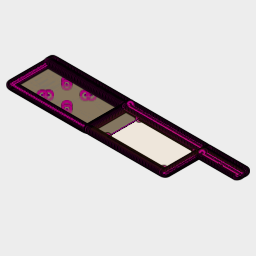
Case v2 (Autodesk Fusion 360 design; units mm, degrees)
Autodesk Fusion 360 part; units mm, degrees
(part 1 of 8)
sketch "Sketch4" plane through (0, 0, 0) normal (0, 1, 0) x (1, 0, 0)
  line L0 (6.35, -6.35) -> (11.1, -6.35)
  line L1 (11.1, -6.35) -> (11.1, -9.35)
  line L2 (11.1, -9.35) -> (15.85, -9.35)
  line L3 (15.85, -9.35) -> (15.85, -6.35)
  line L4 (15.85, -6.35) -> (18.85, -6.35)
  line L5 (18.85, -6.35) -> (18.85, -9.35)
  line L6 (18.85, -9.35) -> (21.85, -9.35)
  line L7 (21.85, -9.35) -> (21.85, -6.35)
  line L8 (21.85, -6.35) -> (24.85, -6.35)
  line L9 (24.85, -6.35) -> (24.85, -9.35)
  line L10 (24.85, -9.35) -> (27.85, -9.35)
  line L11 (27.85, -9.35) -> (27.85, -6.35)
  line L12 (27.85, -6.35) -> (30.85, -6.35)
  line L13 (30.85, -6.35) -> (30.85, -9.35)
  line L14 (30.85, -9.35) -> (33.85, -9.35)
  line L15 (33.85, -9.35) -> (33.85, -6.35)
  line L16 (33.85, -6.35) -> (36.85, -6.35)
  line L17 (36.85, -6.35) -> (36.85, -9.35)
  line L18 (36.85, -9.35) -> (39.85, -9.35)
  line L19 (39.85, -9.35) -> (39.85, -6.35)
  line L20 (39.85, -6.35) -> (42.85, -6.35)
  line L21 (42.85, -6.35) -> (42.85, -9.35)
  line L22 (42.85, -9.35) -> (45.85, -9.35)
  line L23 (45.85, -9.35) -> (45.85, -6.35)
  line L24 (45.85, -6.35) -> (48.85, -6.35)
  line L25 (48.85, -6.35) -> (48.85, -9.35)
  line L26 (48.85, -9.35) -> (51.85, -9.35)
  line L27 (51.85, -9.35) -> (51.85, -6.35)
  line L28 (51.85, -6.35) -> (54.85, -6.35)
  line L29 (54.85, -6.35) -> (54.85, -9.35)
  line L30 (54.85, -9.35) -> (57.85, -9.35)
  line L31 (57.85, -9.35) -> (57.85, -6.35)
  line L32 (57.85, -6.35) -> (60.8501, -6.35)
  line L33 (60.8501, -6.35) -> (60.8501, -9.35)
  line L34 (60.8501, -9.35) -> (63.8501, -9.35)
  line L35 (63.8501, -9.35) -> (63.8501, -6.35)
  line L36 (63.8501, -6.35) -> (66.8501, -6.35)
  line L37 (66.8501, -6.35) -> (66.8501, -9.35)
  line L38 (66.8501, -9.35) -> (69.8501, -9.35)
  line L39 (69.8501, -9.35) -> (69.8501, -6.35)
  line L40 (69.8501, -6.35) -> (72.8501, -6.35)
  line L41 (72.8501, -6.35) -> (72.8501, -9.35)
  line L42 (72.8501, -9.35) -> (75.8501, -9.35)
  line L43 (75.8501, -9.35) -> (75.8501, -6.35)
  line L44 (75.8501, -6.35) -> (78.8501, -6.35)
  line L45 (78.8501, -6.35) -> (78.8501, -9.35)
  line L46 (78.8501, -9.35) -> (81.8501, -9.35)
  line L47 (81.8501, -9.35) -> (81.8501, -6.35)
  line L48 (81.8501, -6.35) -> (84.8501, -6.35)
  line L49 (84.8501, -6.35) -> (84.8501, -9.35)
  line L50 (84.8501, -9.35) -> (87.8501, -9.35)
  line L51 (87.8501, -9.35) -> (87.8501, -6.35)
  line L52 (87.8501, -6.35) -> (90.8501, -6.35)
  line L53 (90.8501, -6.35) -> (90.8501, -9.35)
  line L54 (90.8501, -9.35) -> (93.8501, -9.35)
  line L55 (93.8501, -9.35) -> (93.8501, -6.35)
  line L56 (93.8501, -6.35) -> (96.8501, -6.35)
  line L57 (96.8501, -6.35) -> (96.8501, -9.35)
  line L58 (96.8501, -9.35) -> (99.8501, -9.35)
  line L59 (99.8501, -9.35) -> (99.8501, -6.35)
  line L60 (99.8501, -6.35) -> (102.8501, -6.35)
  line L61 (102.8501, -6.35) -> (102.8501, -9.35)
  line L62 (102.8501, -9.35) -> (105.8501, -9.35)
  line L63 (105.8501, -9.35) -> (105.8501, -6.35)
  line L64 (105.8501, -6.35) -> (108.8501, -6.35)
  line L65 (108.8501, -6.35) -> (108.8501, -9.35)
  line L66 (108.8501, -9.35) -> (111.8501, -9.35)
  line L67 (111.8501, -9.35) -> (111.8501, -6.35)
  line L68 (111.8501, -6.35) -> (114.8501, -6.35)
  line L69 (114.8501, -6.35) -> (114.8501, -9.35)
  line L70 (114.8501, -9.35) -> (117.8501, -9.35)
  line L71 (117.8501, -9.35) -> (117.8501, -6.35)
  line L72 (117.8501, -6.35) -> (120.8501, -6.35)
  line L73 (120.8501, -6.35) -> (120.8501, -9.35)
  line L74 (120.8501, -9.35) -> (123.8501, -9.35)
  line L75 (123.8501, -9.35) -> (123.8501, -6.35)
  line L76 (123.8501, -6.35) -> (126.8501, -6.35)
  line L77 (126.8501, -6.35) -> (126.8501, -9.35)
  line L78 (126.8501, -9.35) -> (129.8501, -9.35)
  line L79 (129.8501, -9.35) -> (129.8501, -6.35)
  line L80 (129.8501, -6.35) -> (132.8501, -6.35)
  line L81 (132.8501, -6.35) -> (132.8501, -9.35)
  line L82 (132.8501, -9.35) -> (135.8501, -9.35)
  line L83 (135.8501, -9.35) -> (135.8501, -6.35)
  line L84 (135.8501, -6.35) -> (138.8501, -6.35)
  line L85 (138.8501, -6.35) -> (138.8501, -9.35)
  line L86 (138.8501, -9.35) -> (141.8501, -9.35)
  line L87 (141.8501, -9.35) -> (141.8501, -6.35)
  line L88 (141.8501, -6.35) -> (144.8501, -6.35)
  line L89 (144.8501, -6.35) -> (144.8501, -9.35)
  line L90 (144.8501, -9.35) -> (147.8501, -9.35)
  line L91 (147.8501, -9.35) -> (147.8501, -6.35)
  line L92 (147.8501, -6.35) -> (150.8501, -6.35)
  line L93 (150.8501, -6.35) -> (150.8501, -9.35)
  line L94 (150.8501, -9.35) -> (153.8501, -9.35)
  line L95 (153.8501, -9.35) -> (153.8501, -6.35)
  line L96 (153.8501, -6.35) -> (156.8501, -6.35)
  line L97 (156.8501, -6.35) -> (156.8501, -9.35)
  line L98 (156.8501, -9.35) -> (159.8501, -9.35)
  line L99 (159.8501, -9.35) -> (159.8501, -6.35)
  line L100 (159.8501, -6.35) -> (162.8501, -6.35)
  line L101 (162.8501, -6.35) -> (162.8501, -9.35)
  line L102 (162.8501, -9.35) -> (165.8501, -9.35)
  line L103 (165.8501, -9.35) -> (165.8501, -6.35)
  line L104 (165.8501, -6.35) -> (168.8501, -6.35)
  line L105 (168.8501, -6.35) -> (168.8501, -9.35)
  line L106 (168.8501, -9.35) -> (171.8501, -9.35)
  line L107 (171.8501, -9.35) -> (171.8501, -6.35)
  line L108 (171.8501, -6.35) -> (174.8501, -6.35)
  line L109 (174.8501, -6.35) -> (174.8501, -9.35)
  line L110 (174.8501, -9.35) -> (177.8501, -9.35)
  line L111 (177.8501, -9.35) -> (177.8501, -6.35)
  line L112 (177.8501, -6.35) -> (180.8501, -6.35)
  line L113 (180.8501, -6.35) -> (180.8501, -9.35)
  line L114 (180.8501, -9.35) -> (183.8502, -9.35)
  line L115 (183.8502, -9.35) -> (183.8502, -6.35)
  line L116 (183.8502, -6.35) -> (186.8502, -6.35)
  line L117 (186.8502, -6.35) -> (186.8502, -9.35)
  line L118 (186.8502, -9.35) -> (189.8502, -9.35)
  line L119 (189.8502, -9.35) -> (189.8502, -6.35)
  line L120 (189.8502, -6.35) -> (192.8502, -6.35)
  line L121 (192.8502, -6.35) -> (192.8502, -9.35)
  line L122 (192.8502, -9.35) -> (195.8502, -9.35)
  line L123 (195.8502, -9.35) -> (195.8502, -6.35)
  line L124 (195.8502, -6.35) -> (198.8502, -6.35)
  line L125 (198.8502, -6.35) -> (198.8502, -9.35)
  line L126 (198.8502, -9.35) -> (201.8502, -9.35)
  line L127 (201.8502, -9.35) -> (201.8502, -6.35)
  line L128 (201.8502, -6.35) -> (204.8502, -6.35)
  line L129 (204.8502, -6.35) -> (204.8502, -9.35)
  line L130 (204.8502, -9.35) -> (207.8502, -9.35)
  line L131 (207.8502, -9.35) -> (207.8502, -6.35)
  line L132 (207.8502, -6.35) -> (210.8502, -6.35)
  line L133 (210.8502, -6.35) -> (210.8502, -9.35)
  line L134 (210.8502, -9.35) -> (213.8502, -9.35)
  line L135 (213.8502, -9.35) -> (213.8502, -6.35)
  line L136 (213.8502, -6.35) -> (216.8502, -6.35)
  line L137 (216.8502, -6.35) -> (216.8502, -9.35)
  line L138 (216.8502, -9.35) -> (219.8502, -9.35)
  line L139 (219.8502, -9.35) -> (219.8502, -6.35)
  line L140 (219.8502, -6.35) -> (222.8502, -6.35)
  line L141 (222.8502, -6.35) -> (222.8502, -9.35)
  line L142 (222.8502, -9.35) -> (225.8502, -9.35)
  line L143 (225.8502, -9.35) -> (225.8502, -6.35)
  line L144 (225.8502, -6.35) -> (228.8502, -6.35)
  line L145 (228.8502, -6.35) -> (228.8502, -9.35)
  line L146 (228.8502, -9.35) -> (231.8502, -9.35)
  line L147 (231.8502, -9.35) -> (231.8502, -6.35)
  line L148 (231.8502, -6.35) -> (234.8502, -6.35)
  line L149 (234.8502, -6.35) -> (234.8502, -9.35)
  line L150 (234.8502, -9.35) -> (237.8502, -9.35)
  line L151 (237.8502, -9.35) -> (237.8502, -6.35)
  line L152 (237.8502, -6.35) -> (240.8502, -6.35)
  line L153 (240.8502, -6.35) -> (240.8502, -9.35)
  line L154 (240.8502, -9.35) -> (243.8502, -9.35)
  line L155 (243.8502, -9.35) -> (243.8502, -6.35)
  line L156 (243.8502, -6.35) -> (246.8502, -6.35)
  line L157 (246.8502, -6.35) -> (246.8502, -9.35)
  line L158 (246.8502, -9.35) -> (249.8502, -9.35)
  line L159 (249.8502, -9.35) -> (249.8502, -6.35)
  line L160 (249.8502, -6.35) -> (252.8502, -6.35)
  line L161 (252.8502, -6.35) -> (252.8502, -9.35)
  line L162 (252.8502, -9.35) -> (255.8502, -9.35)
  line L163 (255.8502, -9.35) -> (255.8502, -6.35)
  line L164 (255.8502, -6.35) -> (258.8502, -6.35)
  line L165 (258.8502, -6.35) -> (258.8502, -9.35)
  line L166 (258.8502, -9.35) -> (261.8502, -9.35)
  line L167 (261.8502, -9.35) -> (261.8502, -6.35)
  line L168 (261.8502, -6.35) -> (264.8502, -6.35)
  line L169 (264.8502, -6.35) -> (264.8502, -9.35)
  line L170 (264.8502, -9.35) -> (267.8502, -9.35)
  line L171 (267.8502, -9.35) -> (267.8502, -6.35)
  line L172 (267.8502, -6.35) -> (270.8502, -6.35)
  line L173 (270.8502, -6.35) -> (270.8502, -9.35)
  line L174 (270.8502, -9.35) -> (273.8502, -9.35)
  line L175 (273.8502, -9.35) -> (273.8502, -6.35)
  line L176 (273.8502, -6.35) -> (276.8502, -6.35)
  line L177 (276.8502, -6.35) -> (276.8502, -9.35)
  line L178 (276.8502, -9.35) -> (279.8502, -9.35)
  line L179 (279.8502, -9.35) -> (279.8502, -6.35)
  line L180 (279.8502, -6.35) -> (282.8502, -6.35)
  line L181 (282.8502, -6.35) -> (282.8502, -9.35)
  line L182 (282.8502, -9.35) -> (285.8502, -9.35)
  line L183 (285.8502, -9.35) -> (285.8502, -6.35)
  line L184 (285.8502, -6.35) -> (288.8502, -6.35)
  line L185 (288.8502, -6.35) -> (288.8502, -9.35)
  line L186 (288.8502, -9.35) -> (291.8502, -9.35)
  line L187 (291.8502, -9.35) -> (291.8502, -6.35)
  line L188 (291.8502, -6.35) -> (294.8502, -6.35)
  line L189 (294.8502, -6.35) -> (294.8502, -9.35)
  line L190 (294.8502, -9.35) -> (297.8502, -9.35)
  line L191 (297.8502, -9.35) -> (297.8502, -6.35)
  line L192 (297.8502, -6.35) -> (300.8502, -6.35)
  line L193 (300.8502, -6.35) -> (300.8502, -9.35)
  line L194 (300.8502, -9.35) -> (303.8502, -9.35)
  line L195 (303.8502, -9.35) -> (303.8502, -6.35)
  line L196 (303.8502, -6.35) -> (306.8503, -6.35)
  line L197 (306.8503, -6.35) -> (306.8503, -9.35)
  line L198 (306.8503, -9.35) -> (309.8503, -9.35)
  line L199 (309.8503, -9.35) -> (309.8503, -6.35)
  line L200 (309.8503, -6.35) -> (312.8503, -6.35)
  line L201 (312.8503, -6.35) -> (312.8503, -9.35)
  line L202 (312.8503, -9.35) -> (317.6003, -9.35)
  line L203 (317.6003, -9.35) -> (317.6003, -6.35)
  line L204 (317.6003, -6.35) -> (322.3503, -6.35)
  line L205 (322.3503, -6.35) -> (322.3503, -10.1)
  line L206 (322.3503, -10.1) -> (319.3503, -10.1)
  line L207 (319.3503, -10.1) -> (319.3503, -13.85)
  line L208 (319.3503, -13.85) -> (322.3503, -13.85)
  line L209 (322.3503, -13.85) -> (322.3503, -16.85)
  line L210 (322.3503, -16.85) -> (319.3503, -16.85)
  line L211 (319.3503, -16.85) -> (319.3503, -20.6)
  line L212 (319.3503, -20.6) -> (322.3503, -20.6)
  line L213 (322.3503, -20.6) -> (322.3503, -24.35)
  line L214 (322.3503, -24.35) -> (317.6003, -24.35)
  line L215 (317.6003, -24.35) -> (317.6003, -21.35)
  line L216 (317.6003, -21.35) -> (312.8503, -21.35)
  line L217 (312.8503, -21.35) -> (312.8503, -24.35)
  line L218 (312.8503, -24.35) -> (309.8503, -24.35)
  line L219 (309.8503, -24.35) -> (309.8503, -21.35)
  line L220 (309.8503, -21.35) -> (306.8503, -21.35)
  line L221 (306.8503, -21.35) -> (306.8503, -24.35)
  line L222 (306.8503, -24.35) -> (303.8502, -24.35)
  line L223 (303.8502, -24.35) -> (303.8502, -21.35)
  line L224 (303.8502, -21.35) -> (300.8502, -21.35)
  line L225 (300.8502, -21.35) -> (300.8502, -24.35)
  line L226 (300.8502, -24.35) -> (297.8502, -24.35)
  line L227 (297.8502, -24.35) -> (297.8502, -21.35)
  line L228 (297.8502, -21.35) -> (294.8502, -21.35)
  line L229 (294.8502, -21.35) -> (294.8502, -24.35)
  line L230 (294.8502, -24.35) -> (291.8502, -24.35)
  line L231 (291.8502, -24.35) -> (291.8502, -21.35)
  line L232 (291.8502, -21.35) -> (288.8502, -21.35)
  line L233 (288.8502, -21.35) -> (288.8502, -24.35)
  line L234 (288.8502, -24.35) -> (285.8502, -24.35)
  line L235 (285.8502, -24.35) -> (285.8502, -21.35)
  line L236 (285.8502, -21.35) -> (282.8502, -21.35)
  line L237 (282.8502, -21.35) -> (282.8502, -24.35)
  line L238 (282.8502, -24.35) -> (279.8502, -24.35)
  line L239 (279.8502, -24.35) -> (279.8502, -21.35)
  line L240 (279.8502, -21.35) -> (276.8502, -21.35)
  line L241 (276.8502, -21.35) -> (276.8502, -24.35)
  line L242 (276.8502, -24.35) -> (273.8502, -24.35)
  line L243 (273.8502, -24.35) -> (273.8502, -21.35)
  line L244 (273.8502, -21.35) -> (270.8502, -21.35)
  line L245 (270.8502, -21.35) -> (270.8502, -24.35)
  line L246 (270.8502, -24.35) -> (267.8502, -24.35)
  line L247 (267.8502, -24.35) -> (267.8502, -21.35)
  line L248 (267.8502, -21.35) -> (264.8502, -21.35)
  line L249 (264.8502, -21.35) -> (264.8502, -24.35)
  line L250 (264.8502, -24.35) -> (261.8502, -24.35)
  line L251 (261.8502, -24.35) -> (261.8502, -21.35)
  line L252 (261.8502, -21.35) -> (258.8502, -21.35)
  line L253 (258.8502, -21.35) -> (258.8502, -24.35)
  line L254 (258.8502, -24.35) -> (255.8502, -24.35)
  line L255 (255.8502, -24.35) -> (255.8502, -21.35)
  line L256 (255.8502, -21.35) -> (252.8502, -21.35)
  line L257 (252.8502, -21.35) -> (252.8502, -24.35)
  line L258 (252.8502, -24.35) -> (249.8502, -24.35)
  line L259 (249.8502, -24.35) -> (249.8502, -21.35)
  line L260 (249.8502, -21.35) -> (246.8502, -21.35)
  line L261 (246.8502, -21.35) -> (246.8502, -24.35)
  line L262 (246.8502, -24.35) -> (243.8502, -24.35)
  line L263 (243.8502, -24.35) -> (243.8502, -21.35)
  line L264 (243.8502, -21.35) -> (240.8502, -21.35)
  line L265 (240.8502, -21.35) -> (240.8502, -24.35)
  line L266 (240.8502, -24.35) -> (237.8502, -24.35)
  line L267 (237.8502, -24.35) -> (237.8502, -21.35)
  line L268 (237.8502, -21.35) -> (234.8502, -21.35)
  line L269 (234.8502, -21.35) -> (234.8502, -24.35)
  line L270 (234.8502, -24.35) -> (231.8502, -24.35)
  line L271 (231.8502, -24.35) -> (231.8502, -21.35)
  line L272 (231.8502, -21.35) -> (228.8502, -21.35)
  line L273 (228.8502, -21.35) -> (228.8502, -24.35)
  line L274 (228.8502, -24.35) -> (225.8502, -24.35)
  line L275 (225.8502, -24.35) -> (225.8502, -21.35)
  line L276 (225.8502, -21.35) -> (222.8502, -21.35)
  line L277 (222.8502, -21.35) -> (222.8502, -24.35)
  line L278 (222.8502, -24.35) -> (219.8502, -24.35)
  line L279 (219.8502, -24.35) -> (219.8502, -21.35)
  line L280 (219.8502, -21.35) -> (216.8502, -21.35)
  line L281 (216.8502, -21.35) -> (216.8502, -24.35)
  line L282 (216.8502, -24.35) -> (213.8502, -24.35)
  line L283 (213.8502, -24.35) -> (213.8502, -21.35)
  line L284 (213.8502, -21.35) -> (210.8502, -21.35)
  line L285 (210.8502, -21.35) -> (210.8502, -24.35)
  line L286 (210.8502, -24.35) -> (207.8502, -24.35)
  line L287 (207.8502, -24.35) -> (207.8502, -21.35)
  line L288 (207.8502, -21.35) -> (204.8502, -21.35)
  line L289 (204.8502, -21.35) -> (204.8502, -24.35)
  line L290 (204.8502, -24.35) -> (201.8502, -24.35)
  line L291 (201.8502, -24.35) -> (201.8502, -21.35)
  line L292 (201.8502, -21.35) -> (198.8502, -21.35)
  line L293 (198.8502, -21.35) -> (198.8502, -24.35)
  line L294 (198.8502, -24.35) -> (195.8502, -24.35)
  line L295 (195.8502, -24.35) -> (195.8502, -21.35)
  line L296 (195.8502, -21.35) -> (192.8502, -21.35)
  line L297 (192.8502, -21.35) -> (192.8502, -24.35)
  line L298 (192.8502, -24.35) -> (189.8502, -24.35)
  line L299 (189.8502, -24.35) -> (189.8502, -21.35)
  line L300 (189.8502, -21.35) -> (186.8502, -21.35)
  line L301 (186.8502, -21.35) -> (186.8502, -24.35)
  line L302 (186.8502, -24.35) -> (183.8502, -24.35)
  line L303 (183.8502, -24.35) -> (183.8502, -21.35)
  line L304 (183.8502, -21.35) -> (180.8501, -21.35)
  line L305 (180.8501, -21.35) -> (180.8501, -24.35)
  line L306 (180.8501, -24.35) -> (177.8501, -24.35)
  line L307 (177.8501, -24.35) -> (177.8501, -21.35)
  line L308 (177.8501, -21.35) -> (174.8501, -21.35)
  line L309 (174.8501, -21.35) -> (174.8501, -24.35)
  line L310 (174.8501, -24.35) -> (171.8501, -24.35)
  line L311 (171.8501, -24.35) -> (171.8501, -21.35)
  line L312 (171.8501, -21.35) -> (168.8501, -21.35)
  line L313 (168.8501, -21.35) -> (168.8501, -24.35)
  line L314 (168.8501, -24.35) -> (165.8501, -24.35)
  line L315 (165.8501, -24.35) -> (165.8501, -21.35)
  line L316 (165.8501, -21.35) -> (162.8501, -21.35)
  line L317 (162.8501, -21.35) -> (162.8501, -24.35)
  line L318 (162.8501, -24.35) -> (159.8501, -24.35)
  line L319 (159.8501, -24.35) -> (159.8501, -21.35)
  line L320 (159.8501, -21.35) -> (156.8501, -21.35)
  line L321 (156.8501, -21.35) -> (156.8501, -24.35)
  line L322 (156.8501, -24.35) -> (153.8501, -24.35)
  line L323 (153.8501, -24.35) -> (153.8501, -21.35)
  line L324 (153.8501, -21.35) -> (150.8501, -21.35)
  line L325 (150.8501, -21.35) -> (150.8501, -24.35)
  line L326 (150.8501, -24.35) -> (147.8501, -24.35)
  line L327 (147.8501, -24.35) -> (147.8501, -21.35)
  line L328 (147.8501, -21.35) -> (144.8501, -21.35)
  line L329 (144.8501, -21.35) -> (144.8501, -24.35)
  line L330 (144.8501, -24.35) -> (141.8501, -24.35)
  line L331 (141.8501, -24.35) -> (141.8501, -21.35)
  line L332 (141.8501, -21.35) -> (138.8501, -21.35)
  line L333 (138.8501, -21.35) -> (138.8501, -24.35)
  line L334 (138.8501, -24.35) -> (135.8501, -24.35)
  line L335 (135.8501, -24.35) -> (135.8501, -21.35)
  line L336 (135.8501, -21.35) -> (132.8501, -21.35)
  line L337 (132.8501, -21.35) -> (132.8501, -24.35)
  line L338 (132.8501, -24.35) -> (129.8501, -24.35)
  line L339 (129.8501, -24.35) -> (129.8501, -21.35)
  line L340 (129.8501, -21.35) -> (126.8501, -21.35)
  line L341 (126.8501, -21.35) -> (126.8501, -24.35)
  line L342 (126.8501, -24.35) -> (123.8501, -24.35)
  line L343 (123.8501, -24.35) -> (123.8501, -21.35)
  line L344 (123.8501, -21.35) -> (120.8501, -21.35)
  line L345 (120.8501, -21.35) -> (120.8501, -24.35)
  line L346 (120.8501, -24.35) -> (117.8501, -24.35)
  line L347 (117.8501, -24.35) -> (117.8501, -21.35)
  line L348 (117.8501, -21.35) -> (114.8501, -21.35)
  line L349 (114.8501, -21.35) -> (114.8501, -24.35)
  line L350 (114.8501, -24.35) -> (111.8501, -24.35)
  line L351 (111.8501, -24.35) -> (111.8501, -21.35)
  line L352 (111.8501, -21.35) -> (108.8501, -21.35)
  line L353 (108.8501, -21.35) -> (108.8501, -24.35)
  line L354 (108.8501, -24.35) -> (105.8501, -24.35)
  line L355 (105.8501, -24.35) -> (105.8501, -21.35)
  line L356 (105.8501, -21.35) -> (102.8501, -21.35)
  line L357 (102.8501, -21.35) -> (102.8501, -24.35)
  line L358 (102.8501, -24.35) -> (99.8501, -24.35)
  line L359 (99.8501, -24.35) -> (99.8501, -21.35)
  line L360 (99.8501, -21.35) -> (96.8501, -21.35)
  line L361 (96.8501, -21.35) -> (96.8501, -24.35)
  line L362 (96.8501, -24.35) -> (93.8501, -24.35)
  line L363 (93.8501, -24.35) -> (93.8501, -21.35)
  line L364 (93.8501, -21.35) -> (90.8501, -21.35)
  line L365 (90.8501, -21.35) -> (90.8501, -24.35)
  line L366 (90.8501, -24.35) -> (87.8501, -24.35)
  line L367 (87.8501, -24.35) -> (87.8501, -21.35)
  line L368 (87.8501, -21.35) -> (84.8501, -21.35)
  line L369 (84.8501, -21.35) -> (84.8501, -24.35)
  line L370 (84.8501, -24.35) -> (81.8501, -24.35)
  line L371 (81.8501, -24.35) -> (81.8501, -21.35)
  line L372 (81.8501, -21.35) -> (78.8501, -21.35)
  line L373 (78.8501, -21.35) -> (78.8501, -24.35)
  line L374 (78.8501, -24.35) -> (75.8501, -24.35)
  line L375 (75.8501, -24.35) -> (75.8501, -21.35)
  line L376 (75.8501, -21.35) -> (72.8501, -21.35)
  line L377 (72.8501, -21.35) -> (72.8501, -24.35)
  line L378 (72.8501, -24.35) -> (69.8501, -24.35)
  line L379 (69.8501, -24.35) -> (69.8501, -21.35)
  line L380 (69.8501, -21.35) -> (66.8501, -21.35)
  line L381 (66.8501, -21.35) -> (66.8501, -24.35)
  line L382 (66.8501, -24.35) -> (63.8501, -24.35)
  line L383 (63.8501, -24.35) -> (63.8501, -21.35)
  line L384 (63.8501, -21.35) -> (60.8501, -21.35)
  line L385 (60.8501, -21.35) -> (60.8501, -24.35)
  line L386 (60.8501, -24.35) -> (57.85, -24.35)
  line L387 (57.85, -24.35) -> (57.85, -21.35)
  line L388 (57.85, -21.35) -> (54.85, -21.35)
  line L389 (54.85, -21.35) -> (54.85, -24.35)
  line L390 (54.85, -24.35) -> (51.85, -24.35)
  line L391 (51.85, -24.35) -> (51.85, -21.35)
  line L392 (51.85, -21.35) -> (48.85, -21.35)
  line L393 (48.85, -21.35) -> (48.85, -24.35)
  line L394 (48.85, -24.35) -> (45.85, -24.35)
  line L395 (45.85, -24.35) -> (45.85, -21.35)
  line L396 (45.85, -21.35) -> (42.85, -21.35)
  line L397 (42.85, -21.35) -> (42.85, -24.35)
  line L398 (42.85, -24.35) -> (39.85, -24.35)
  line L399 (39.85, -24.35) -> (39.85, -21.35)
  line L400 (39.85, -21.35) -> (36.85, -21.35)
  line L401 (36.85, -21.35) -> (36.85, -24.35)
  line L402 (36.85, -24.35) -> (33.85, -24.35)
  line L403 (33.85, -24.35) -> (33.85, -21.35)
  line L404 (33.85, -21.35) -> (30.85, -21.35)
  line L405 (30.85, -21.35) -> (30.85, -24.35)
  line L406 (30.85, -24.35) -> (27.85, -24.35)
  line L407 (27.85, -24.35) -> (27.85, -21.35)
  line L408 (27.85, -21.35) -> (24.85, -21.35)
  line L409 (24.85, -21.35) -> (24.85, -24.35)
  line L410 (24.85, -24.35) -> (21.85, -24.35)
  line L411 (21.85, -24.35) -> (21.85, -21.35)
  line L412 (21.85, -21.35) -> (18.85, -21.35)
  line L413 (18.85, -21.35) -> (18.85, -24.35)
  line L414 (18.85, -24.35) -> (15.85, -24.35)
  line L415 (15.85, -24.35) -> (15.85, -21.35)
  line L416 (15.85, -21.35) -> (11.1, -21.35)
  line L417 (11.1, -21.35) -> (11.1, -24.35)
  line L418 (11.1, -24.35) -> (6.35, -24.35)
  line L419 (6.35, -24.35) -> (6.35, -20.6)
  line L420 (6.35, -20.6) -> (9.35, -20.6)
  line L421 (9.35, -20.6) -> (9.35, -16.85)
  line L422 (9.35, -16.85) -> (6.35, -16.85)
  line L423 (6.35, -16.85) -> (6.35, -13.85)
  line L424 (6.35, -13.85) -> (9.35, -13.85)
  line L425 (9.35, -13.85) -> (9.35, -10.1)
  line L426 (9.35, -10.1) -> (6.35, -10.1)
  line L427 (6.35, -10.1) -> (6.35, -6.35)
  line L428 (322.3503, -6.35) -> (327.1003, -6.35)
  line L429 (327.1003, -6.35) -> (327.1003, -9.35)
  line L430 (327.1003, -9.35) -> (331.8503, -9.35)
  line L431 (331.8503, -9.35) -> (331.8503, -6.35)
  line L432 (331.8503, -6.35) -> (334.8503, -6.35)
  line L433 (334.8503, -6.35) -> (334.8503, -9.35)
  line L434 (334.8503, -9.35) -> (337.8503, -9.35)
  line L435 (337.8503, -9.35) -> (337.8503, -6.35)
  line L436 (337.8503, -6.35) -> (340.8503, -6.35)
  line L437 (340.8503, -6.35) -> (340.8503, -9.35)
  line L438 (340.8503, -9.35) -> (343.8503, -9.35)
  line L439 (343.8503, -9.35) -> (343.8503, -6.35)
  line L440 (343.8503, -6.35) -> (346.8503, -6.35)
  line L441 (346.8503, -6.35) -> (346.8503, -9.35)
  line L442 (346.8503, -9.35) -> (349.8503, -9.35)
  line L443 (349.8503, -9.35) -> (349.8503, -6.35)
  line L444 (349.8503, -6.35) -> (352.8503, -6.35)
  line L445 (352.8503, -6.35) -> (352.8503, -9.35)
  line L446 (352.8503, -9.35) -> (355.8503, -9.35)
  line L447 (355.8503, -9.35) -> (355.8503, -6.35)
  line L448 (355.8503, -6.35) -> (358.8503, -6.35)
  line L449 (358.8503, -6.35) -> (358.8503, -9.35)
  line L450 (358.8503, -9.35) -> (361.8503, -9.35)
  line L451 (361.8503, -9.35) -> (361.8503, -6.35)
  line L452 (361.8503, -6.35) -> (364.8503, -6.35)
  line L453 (364.8503, -6.35) -> (364.8503, -9.35)
  line L454 (364.8503, -9.35) -> (367.8503, -9.35)
  line L455 (367.8503, -9.35) -> (367.8503, -6.35)
  line L456 (367.8503, -6.35) -> (370.8503, -6.35)
  line L457 (370.8503, -6.35) -> (370.8503, -9.35)
  line L458 (370.8503, -9.35) -> (373.8503, -9.35)
  line L459 (373.8503, -9.35) -> (373.8503, -6.35)
  line L460 (373.8503, -6.35) -> (376.8503, -6.35)
  line L461 (376.8503, -6.35) -> (376.8503, -9.35)
  line L462 (376.8503, -9.35) -> (379.8503, -9.35)
  line L463 (379.8503, -9.35) -> (379.8503, -6.35)
  line L464 (379.8503, -6.35) -> (382.8503, -6.35)
  line L465 (382.8503, -6.35) -> (382.8503, -9.35)
  line L466 (382.8503, -9.35) -> (385.8503, -9.35)
  line L467 (385.8503, -9.35) -> (385.8503, -6.35)
  line L468 (385.8503, -6.35) -> (388.8503, -6.35)
  line L469 (388.8503, -6.35) -> (388.8503, -9.35)
  line L470 (388.8503, -9.35) -> (391.8503, -9.35)
  line L471 (391.8503, -9.35) -> (391.8503, -6.35)
  line L472 (391.8503, -6.35) -> (394.8503, -6.35)
  line L473 (394.8503, -6.35) -> (394.8503, -9.35)
  line L474 (394.8503, -9.35) -> (397.8503, -9.35)
  line L475 (397.8503, -9.35) -> (397.8503, -6.35)
  line L476 (397.8503, -6.35) -> (400.8503, -6.35)
  line L477 (400.8503, -6.35) -> (400.8503, -9.35)
  line L478 (400.8503, -9.35) -> (403.8503, -9.35)
  line L479 (403.8503, -9.35) -> (403.8503, -6.35)
  line L480 (403.8503, -6.35) -> (406.8503, -6.35)
  line L481 (406.8503, -6.35) -> (406.8503, -9.35)
  line L482 (406.8503, -9.35) -> (409.8503, -9.35)
  line L483 (409.8503, -9.35) -> (409.8503, -6.35)
  line L484 (409.8503, -6.35) -> (412.8503, -6.35)
  line L485 (412.8503, -6.35) -> (412.8503, -9.35)
  line L486 (412.8503, -9.35) -> (415.8503, -9.35)
  line L487 (415.8503, -9.35) -> (415.8503, -6.35)
  line L488 (415.8503, -6.35) -> (418.8503, -6.35)
  line L489 (418.8503, -6.35) -> (418.8503, -9.35)
  line L490 (418.8503, -9.35) -> (421.8503, -9.35)
  line L491 (421.8503, -9.35) -> (421.8503, -6.35)
  line L492 (421.8503, -6.35) -> (424.8503, -6.35)
  line L493 (424.8503, -6.35) -> (424.8503, -9.35)
  line L494 (424.8503, -9.35) -> (427.8504, -9.35)
  line L495 (427.8504, -9.35) -> (427.8504, -6.35)
  line L496 (427.8504, -6.35) -> (430.8504, -6.35)
  line L497 (430.8504, -6.35) -> (430.8504, -9.35)
  line L498 (430.8504, -9.35) -> (433.8504, -9.35)
  line L499 (433.8504, -9.35) -> (433.8504, -6.35)
  line L500 (433.8504, -6.35) -> (436.8504, -6.35)
  line L501 (436.8504, -6.35) -> (436.8504, -9.35)
  line L502 (436.8504, -9.35) -> (439.8504, -9.35)
  line L503 (439.8504, -9.35) -> (439.8504, -6.35)
  line L504 (439.8504, -6.35) -> (442.8504, -6.35)
  line L505 (442.8504, -6.35) -> (442.8504, -9.35)
  line L506 (442.8504, -9.35) -> (445.8504, -9.35)
  line L507 (445.8504, -9.35) -> (445.8504, -6.35)
  line L508 (445.8504, -6.35) -> (448.8504, -6.35)
  line L509 (448.8504, -6.35) -> (448.8504, -9.35)
  line L510 (448.8504, -9.35) -> (451.8504, -9.35)
  line L511 (451.8504, -9.35) -> (451.8504, -6.35)
  line L512 (451.8504, -6.35) -> (454.8504, -6.35)
  line L513 (454.8504, -6.35) -> (454.8504, -9.35)
  line L514 (454.8504, -9.35) -> (457.8504, -9.35)
  line L515 (457.8504, -9.35) -> (457.8504, -6.35)
  line L516 (457.8504, -6.35) -> (460.8504, -6.35)
  line L517 (460.8504, -6.35) -> (460.8504, -9.35)
  line L518 (460.8504, -9.35) -> (463.8504, -9.35)
  line L519 (463.8504, -9.35) -> (463.8504, -6.35)
  line L520 (463.8504, -6.35) -> (466.8504, -6.35)
  line L521 (466.8504, -6.35) -> (466.8504, -9.35)
  line L522 (466.8504, -9.35) -> (469.8504, -9.35)
  line L523 (469.8504, -9.35) -> (469.8504, -6.35)
  line L524 (469.8504, -6.35) -> (472.8504, -6.35)
  line L525 (472.8504, -6.35) -> (472.8504, -9.35)
  line L526 (472.8504, -9.35) -> (475.8504, -9.35)
  line L527 (475.8504, -9.35) -> (475.8504, -6.35)
  line L528 (475.8504, -6.35) -> (478.8504, -6.35)
  line L529 (478.8504, -6.35) -> (478.8504, -9.35)
  line L530 (478.8504, -9.35) -> (481.8504, -9.35)
  line L531 (481.8504, -9.35) -> (481.8504, -6.35)
  line L532 (481.8504, -6.35) -> (484.8504, -6.35)
  line L533 (484.8504, -6.35) -> (484.8504, -9.35)
  line L534 (484.8504, -9.35) -> (487.8504, -9.35)
  line L535 (487.8504, -9.35) -> (487.8504, -6.35)
  line L536 (487.8504, -6.35) -> (490.8504, -6.35)
  line L537 (490.8504, -6.35) -> (490.8504, -9.35)
  line L538 (490.8504, -9.35) -> (493.8504, -9.35)
  line L539 (493.8504, -9.35) -> (493.8504, -6.35)
  line L540 (493.8504, -6.35) -> (496.8504, -6.35)
  line L541 (496.8504, -6.35) -> (496.8504, -9.35)
  line L542 (496.8504, -9.35) -> (499.8504, -9.35)
  line L543 (499.8504, -9.35) -> (499.8504, -6.35)
  line L544 (499.8504, -6.35) -> (502.8504, -6.35)
  line L545 (502.8504, -6.35) -> (502.8504, -9.35)
  line L546 (502.8504, -9.35) -> (505.8504, -9.35)
  line L547 (505.8504, -9.35) -> (505.8504, -6.35)
  line L548 (505.8504, -6.35) -> (508.8504, -6.35)
  line L549 (508.8504, -6.35) -> (508.8504, -9.35)
  line L550 (508.8504, -9.35) -> (511.8504, -9.35)
  line L551 (511.8504, -9.35) -> (511.8504, -6.35)
  line L552 (511.8504, -6.35) -> (514.8504, -6.35)
  line L553 (514.8504, -6.35) -> (514.8504, -9.35)
  line L554 (514.8504, -9.35) -> (517.8504, -9.35)
  line L555 (517.8504, -9.35) -> (517.8504, -6.35)
  line L556 (517.8504, -6.35) -> (520.8504, -6.35)
  line L557 (520.8504, -6.35) -> (520.8504, -9.35)
  line L558 (520.8504, -9.35) -> (523.8504, -9.35)
  line L559 (523.8504, -9.35) -> (523.8504, -6.35)
  line L560 (523.8504, -6.35) -> (526.8504, -6.35)
  line L561 (526.8504, -6.35) -> (526.8504, -9.35)
  line L562 (526.8504, -9.35) -> (529.8504, -9.35)
  line L563 (529.8504, -9.35) -> (529.8504, -6.35)
  line L564 (529.8504, -6.35) -> (532.8504, -6.35)
  line L565 (532.8504, -6.35) -> (532.8504, -9.35)
  line L566 (532.8504, -9.35) -> (535.8504, -9.35)
  line L567 (535.8504, -9.35) -> (535.8504, -6.35)
  line L568 (535.8504, -6.35) -> (538.8504, -6.35)
  line L569 (538.8504, -6.35) -> (538.8504, -9.35)
  line L570 (538.8504, -9.35) -> (541.8504, -9.35)
  line L571 (541.8504, -9.35) -> (541.8504, -6.35)
  line L572 (541.8504, -6.35) -> (544.8504, -6.35)
  line L573 (544.8504, -6.35) -> (544.8504, -9.35)
  line L574 (544.8504, -9.35) -> (547.8505, -9.35)
  line L575 (547.8505, -9.35) -> (547.8505, -6.35)
  line L576 (547.8505, -6.35) -> (550.8505, -6.35)
  line L577 (550.8505, -6.35) -> (550.8505, -9.35)
  line L578 (550.8505, -9.35) -> (553.8505, -9.35)
  line L579 (553.8505, -9.35) -> (553.8505, -6.35)
  line L580 (553.8505, -6.35) -> (556.8505, -6.35)
  line L581 (556.8505, -6.35) -> (556.8505, -9.35)
  line L582 (556.8505, -9.35) -> (559.8505, -9.35)
  line L583 (559.8505, -9.35) -> (559.8505, -6.35)
  line L584 (559.8505, -6.35) -> (562.8505, -6.35)
  line L585 (562.8505, -6.35) -> (562.8505, -9.35)
  line L586 (562.8505, -9.35) -> (565.8505, -9.35)
  line L587 (565.8505, -9.35) -> (565.8505, -6.35)
  line L588 (565.8505, -6.35) -> (568.8505, -6.35)
  line L589 (568.8505, -6.35) -> (568.8505, -9.35)
  line L590 (568.8505, -9.35) -> (571.8505, -9.35)
  line L591 (571.8505, -9.35) -> (571.8505, -6.35)
  line L592 (571.8505, -6.35) -> (574.8505, -6.35)
  line L593 (574.8505, -6.35) -> (574.8505, -9.35)
  line L594 (574.8505, -9.35) -> (577.8505, -9.35)
  line L595 (577.8505, -9.35) -> (577.8505, -6.35)
  line L596 (577.8505, -6.35) -> (580.8505, -6.35)
  line L597 (580.8505, -6.35) -> (580.8505, -9.35)
  line L598 (580.8505, -9.35) -> (583.8505, -9.35)
  line L599 (583.8505, -9.35) -> (583.8505, -6.35)
  line L600 (583.8505, -6.35) -> (586.8505, -6.35)
  line L601 (586.8505, -6.35) -> (586.8505, -9.35)
  line L602 (586.8505, -9.35) -> (589.8505, -9.35)
  line L603 (589.8505, -9.35) -> (589.8505, -6.35)
  line L604 (589.8505, -6.35) -> (592.8505, -6.35)
  line L605 (592.8505, -6.35) -> (592.8505, -9.35)
  line L606 (592.8505, -9.35) -> (595.8505, -9.35)
  line L607 (595.8505, -9.35) -> (595.8505, -6.35)
  line L608 (595.8505, -6.35) -> (598.8505, -6.35)
  line L609 (598.8505, -6.35) -> (598.8505, -9.35)
  line L610 (598.8505, -9.35) -> (601.8505, -9.35)
  line L611 (601.8505, -9.35) -> (601.8505, -6.35)
  line L612 (601.8505, -6.35) -> (604.8505, -6.35)
  line L613 (604.8505, -6.35) -> (604.8505, -9.35)
  line L614 (604.8505, -9.35) -> (607.8505, -9.35)
  line L615 (607.8505, -9.35) -> (607.8505, -6.35)
  line L616 (607.8505, -6.35) -> (610.8505, -6.35)
  line L617 (610.8505, -6.35) -> (610.8505, -9.35)
  line L618 (610.8505, -9.35) -> (613.8505, -9.35)
  line L619 (613.8505, -9.35) -> (613.8505, -6.35)
  line L620 (613.8505, -6.35) -> (616.8505, -6.35)
  line L621 (616.8505, -6.35) -> (616.8505, -9.35)
  line L622 (616.8505, -9.35) -> (619.8505, -9.35)
  line L623 (619.8505, -9.35) -> (619.8505, -6.35)
  line L624 (619.8505, -6.35) -> (622.8505, -6.35)
  line L625 (622.8505, -6.35) -> (622.8505, -9.35)
  line L626 (622.8505, -9.35) -> (625.8505, -9.35)
  line L627 (625.8505, -9.35) -> (625.8505, -6.35)
  line L628 (625.8505, -6.35) -> (628.8505, -6.35)
  line L629 (628.8505, -6.35) -> (628.8505, -9.35)
  line L630 (628.8505, -9.35) -> (633.6005, -9.35)
  line L631 (633.6005, -9.35) -> (633.6005, -6.35)
  line L632 (633.6005, -6.35) -> (638.3505, -6.35)
  line L633 (638.3505, -6.35) -> (638.3505, -10.1)
  line L634 (638.3505, -10.1) -> (635.3505, -10.1)
  line L635 (635.3505, -10.1) -> (635.3505, -13.85)
  line L636 (635.3505, -13.85) -> (638.3505, -13.85)
  line L637 (638.3505, -13.85) -> (638.3505, -16.85)
  line L638 (638.3505, -16.85) -> (635.3505, -16.85)
  line L639 (635.3505, -16.85) -> (635.3505, -20.6)
  line L640 (635.3505, -20.6) -> (638.3505, -20.6)
  line L641 (638.3505, -20.6) -> (638.3505, -24.35)
  line L642 (638.3505, -24.35) -> (633.6005, -24.35)
  line L643 (633.6005, -24.35) -> (633.6005, -21.35)
  line L644 (633.6005, -21.35) -> (628.8505, -21.35)
  line L645 (628.8505, -21.35) -> (628.8505, -24.35)
  line L646 (628.8505, -24.35) -> (625.8505, -24.35)
  line L647 (625.8505, -24.35) -> (625.8505, -21.35)
  line L648 (625.8505, -21.35) -> (622.8505, -21.35)
  line L649 (622.8505, -21.35) -> (622.8505, -24.35)
  line L650 (622.8505, -24.35) -> (619.8505, -24.35)
  line L651 (619.8505, -24.35) -> (619.8505, -21.35)
  line L652 (619.8505, -21.35) -> (616.8505, -21.35)
  line L653 (616.8505, -21.35) -> (616.8505, -24.35)
  line L654 (616.8505, -24.35) -> (613.8505, -24.35)
  line L655 (613.8505, -24.35) -> (613.8505, -21.35)
  line L656 (613.8505, -21.35) -> (610.8505, -21.35)
  line L657 (610.8505, -21.35) -> (610.8505, -24.35)
  line L658 (610.8505, -24.35) -> (607.8505, -24.35)
  line L659 (607.8505, -24.35) -> (607.8505, -21.35)
  line L660 (607.8505, -21.35) -> (604.8505, -21.35)
  line L661 (604.8505, -21.35) -> (604.8505, -24.35)
  line L662 (604.8505, -24.35) -> (601.8505, -24.35)
  line L663 (601.8505, -24.35) -> (601.8505, -21.35)
  line L664 (601.8505, -21.35) -> (598.8505, -21.35)
  line L665 (598.8505, -21.35) -> (598.8505, -24.35)
  line L666 (598.8505, -24.35) -> (595.8505, -24.35)
  line L667 (595.8505, -24.35) -> (595.8505, -21.35)
  line L668 (595.8505, -21.35) -> (592.8505, -21.35)
  line L669 (592.8505, -21.35) -> (592.8505, -24.35)
  line L670 (592.8505, -24.35) -> (589.8505, -24.35)
  line L671 (589.8505, -24.35) -> (589.8505, -21.35)
  line L672 (589.8505, -21.35) -> (586.8505, -21.35)
  line L673 (586.8505, -21.35) -> (586.8505, -24.35)
  line L674 (586.8505, -24.35) -> (583.8505, -24.35)
  line L675 (583.8505, -24.35) -> (583.8505, -21.35)
  line L676 (583.8505, -21.35) -> (580.8505, -21.35)
  line L677 (580.8505, -21.35) -> (580.8505, -24.35)
  line L678 (580.8505, -24.35) -> (577.8505, -24.35)
  line L679 (577.8505, -24.35) -> (577.8505, -21.35)
  line L680 (577.8505, -21.35) -> (574.8505, -21.35)
  line L681 (574.8505, -21.35) -> (574.8505, -24.35)
  line L682 (574.8505, -24.35) -> (571.8505, -24.35)
  line L683 (571.8505, -24.35) -> (571.8505, -21.35)
  line L684 (571.8505, -21.35) -> (568.8505, -21.35)
  line L685 (568.8505, -21.35) -> (568.8505, -24.35)
  line L686 (568.8505, -24.35) -> (565.8505, -24.35)
  line L687 (565.8505, -24.35) -> (565.8505, -21.35)
  line L688 (565.8505, -21.35) -> (562.8505, -21.35)
  line L689 (562.8505, -21.35) -> (562.8505, -24.35)
  line L690 (562.8505, -24.35) -> (559.8505, -24.35)
  line L691 (559.8505, -24.35) -> (559.8505, -21.35)
  line L692 (559.8505, -21.35) -> (556.8505, -21.35)
  line L693 (556.8505, -21.35) -> (556.8505, -24.35)
  line L694 (556.8505, -24.35) -> (553.8505, -24.35)
  line L695 (553.8505, -24.35) -> (553.8505, -21.35)
  line L696 (553.8505, -21.35) -> (550.8505, -21.35)
  line L697 (550.8505, -21.35) -> (550.8505, -24.35)
  line L698 (550.8505, -24.35) -> (547.8505, -24.35)
  line L699 (547.8505, -24.35) -> (547.8505, -21.35)
  line L700 (547.8505, -21.35) -> (544.8504, -21.35)
  line L701 (544.8504, -21.35) -> (544.8504, -24.35)
  line L702 (544.8504, -24.35) -> (541.8504, -24.35)
  line L703 (541.8504, -24.35) -> (541.8504, -21.35)
  line L704 (541.8504, -21.35) -> (538.8504, -21.35)
  line L705 (538.8504, -21.35) -> (538.8504, -24.35)
  line L706 (538.8504, -24.35) -> (535.8504, -24.35)
  line L707 (535.8504, -24.35) -> (535.8504, -21.35)
  line L708 (535.8504, -21.35) -> (532.8504, -21.35)
  line L709 (532.8504, -21.35) -> (532.8504, -24.35)
  line L710 (532.8504, -24.35) -> (529.8504, -24.35)
  line L711 (529.8504, -24.35) -> (529.8504, -21.35)
  line L712 (529.8504, -21.35) -> (526.8504, -21.35)
  line L713 (526.8504, -21.35) -> (526.8504, -24.35)
  line L714 (526.8504, -24.35) -> (523.8504, -24.35)
  line L715 (523.8504, -24.35) -> (523.8504, -21.35)
  line L716 (523.8504, -21.35) -> (520.8504, -21.35)
  line L717 (520.8504, -21.35) -> (520.8504, -24.35)
  line L718 (520.8504, -24.35) -> (517.8504, -24.35)
  line L719 (517.8504, -24.35) -> (517.8504, -21.35)
  line L720 (517.8504, -21.35) -> (514.8504, -21.35)
  line L721 (514.8504, -21.35) -> (514.8504, -24.35)
  line L722 (514.8504, -24.35) -> (511.8504, -24.35)
  line L723 (511.8504, -24.35) -> (511.8504, -21.35)
  line L724 (511.8504, -21.35) -> (508.8504, -21.35)
  line L725 (508.8504, -21.35) -> (508.8504, -24.35)
  line L726 (508.8504, -24.35) -> (505.8504, -24.35)
  line L727 (505.8504, -24.35) -> (505.8504, -21.35)
  line L728 (505.8504, -21.35) -> (502.8504, -21.35)
  line L729 (502.8504, -21.35) -> (502.8504, -24.35)
  line L730 (502.8504, -24.35) -> (499.8504, -24.35)
  line L731 (499.8504, -24.35) -> (499.8504, -21.35)
  line L732 (499.8504, -21.35) -> (496.8504, -21.35)
  line L733 (496.8504, -21.35) -> (496.8504, -24.35)
  line L734 (496.8504, -24.35) -> (493.8504, -24.35)
  line L735 (493.8504, -24.35) -> (493.8504, -21.35)
  line L736 (493.8504, -21.35) -> (490.8504, -21.35)
  line L737 (490.8504, -21.35) -> (490.8504, -24.35)
  line L738 (490.8504, -24.35) -> (487.8504, -24.35)
  line L739 (487.8504, -24.35) -> (487.8504, -21.35)
  line L740 (487.8504, -21.35) -> (484.8504, -21.35)
  line L741 (484.8504, -21.35) -> (484.8504, -24.35)
  line L742 (484.8504, -24.35) -> (481.8504, -24.35)
  line L743 (481.8504, -24.35) -> (481.8504, -21.35)
  line L744 (481.8504, -21.35) -> (478.8504, -21.35)
  line L745 (478.8504, -21.35) -> (478.8504, -24.35)
  line L746 (478.8504, -24.35) -> (475.8504, -24.35)
  line L747 (475.8504, -24.35) -> (475.8504, -21.35)
  line L748 (475.8504, -21.35) -> (472.8504, -21.35)
  line L749 (472.8504, -21.35) -> (472.8504, -24.35)
  line L750 (472.8504, -24.35) -> (469.8504, -24.35)
  line L751 (469.8504, -24.35) -> (469.8504, -21.35)
  line L752 (469.8504, -21.35) -> (466.8504, -21.35)
  line L753 (466.8504, -21.35) -> (466.8504, -24.35)
  line L754 (466.8504, -24.35) -> (463.8504, -24.35)
  line L755 (463.8504, -24.35) -> (463.8504, -21.35)
  line L756 (463.8504, -21.35) -> (460.8504, -21.35)
  line L757 (460.8504, -21.35) -> (460.8504, -24.35)
  line L758 (460.8504, -24.35) -> (457.8504, -24.35)
  line L759 (457.8504, -24.35) -> (457.8504, -21.35)
  line L760 (457.8504, -21.35) -> (454.8504, -21.35)
  line L761 (454.8504, -21.35) -> (454.8504, -24.35)
  line L762 (454.8504, -24.35) -> (451.8504, -24.35)
  line L763 (451.8504, -24.35) -> (451.8504, -21.35)
  line L764 (451.8504, -21.35) -> (448.8504, -21.35)
  line L765 (448.8504, -21.35) -> (448.8504, -24.35)
  line L766 (448.8504, -24.35) -> (445.8504, -24.35)
  line L767 (445.8504, -24.35) -> (445.8504, -21.35)
  line L768 (445.8504, -21.35) -> (442.8504, -21.35)
  line L769 (442.8504, -21.35) -> (442.8504, -24.35)
  line L770 (442.8504, -24.35) -> (439.8504, -24.35)
  line L771 (439.8504, -24.35) -> (439.8504, -21.35)
  line L772 (439.8504, -21.35) -> (436.8504, -21.35)
  line L773 (436.8504, -21.35) -> (436.8504, -24.35)
  line L774 (436.8504, -24.35) -> (433.8504, -24.35)
  line L775 (433.8504, -24.35) -> (433.8504, -21.35)
  line L776 (433.8504, -21.35) -> (430.8504, -21.35)
  line L777 (430.8504, -21.35) -> (430.8504, -24.35)
  line L778 (430.8504, -24.35) -> (427.8504, -24.35)
  line L779 (427.8504, -24.35) -> (427.8504, -21.35)
  line L780 (427.8504, -21.35) -> (424.8503, -21.35)
  line L781 (424.8503, -21.35) -> (424.8503, -24.35)
  line L782 (424.8503, -24.35) -> (421.8503, -24.35)
  line L783 (421.8503, -24.35) -> (421.8503, -21.35)
  line L784 (421.8503, -21.35) -> (418.8503, -21.35)
  line L785 (418.8503, -21.35) -> (418.8503, -24.35)
  line L786 (418.8503, -24.35) -> (415.8503, -24.35)
  line L787 (415.8503, -24.35) -> (415.8503, -21.35)
  line L788 (415.8503, -21.35) -> (412.8503, -21.35)
  line L789 (412.8503, -21.35) -> (412.8503, -24.35)
  line L790 (412.8503, -24.35) -> (409.8503, -24.35)
  line L791 (409.8503, -24.35) -> (409.8503, -21.35)
  line L792 (409.8503, -21.35) -> (406.8503, -21.35)
  line L793 (406.8503, -21.35) -> (406.8503, -24.35)
  line L794 (406.8503, -24.35) -> (403.8503, -24.35)
  line L795 (403.8503, -24.35) -> (403.8503, -21.35)
  line L796 (403.8503, -21.35) -> (400.8503, -21.35)
  line L797 (400.8503, -21.35) -> (400.8503, -24.35)
  line L798 (400.8503, -24.35) -> (397.8503, -24.35)
  line L799 (397.8503, -24.35) -> (397.8503, -21.35)
  line L800 (397.8503, -21.35) -> (394.8503, -21.35)
  line L801 (394.8503, -21.35) -> (394.8503, -24.35)
  line L802 (394.8503, -24.35) -> (391.8503, -24.35)
  line L803 (391.8503, -24.35) -> (391.8503, -21.35)
  line L804 (391.8503, -21.35) -> (388.8503, -21.35)
  line L805 (388.8503, -21.35) -> (388.8503, -24.35)
  line L806 (388.8503, -24.35) -> (385.8503, -24.35)
  line L807 (385.8503, -24.35) -> (385.8503, -21.35)
  line L808 (385.8503, -21.35) -> (382.8503, -21.35)
  line L809 (382.8503, -21.35) -> (382.8503, -24.35)
  line L810 (382.8503, -24.35) -> (379.8503, -24.35)
  line L811 (379.8503, -24.35) -> (379.8503, -21.35)
  line L812 (379.8503, -21.35) -> (376.8503, -21.35)
  line L813 (376.8503, -21.35) -> (376.8503, -24.35)
  line L814 (376.8503, -24.35) -> (373.8503, -24.35)
  line L815 (373.8503, -24.35) -> (373.8503, -21.35)
  line L816 (373.8503, -21.35) -> (370.8503, -21.35)
  line L817 (370.8503, -21.35) -> (370.8503, -24.35)
  line L818 (370.8503, -24.35) -> (367.8503, -24.35)
  line L819 (367.8503, -24.35) -> (367.8503, -21.35)
  line L820 (367.8503, -21.35) -> (364.8503, -21.35)
  line L821 (364.8503, -21.35) -> (364.8503, -24.35)
  line L822 (364.8503, -24.35) -> (361.8503, -24.35)
  line L823 (361.8503, -24.35) -> (361.8503, -21.35)
  line L824 (361.8503, -21.35) -> (358.8503, -21.35)
  line L825 (358.8503, -21.35) -> (358.8503, -24.35)
  line L826 (358.8503, -24.35) -> (355.8503, -24.35)
  line L827 (355.8503, -24.35) -> (355.8503, -21.35)
  line L828 (355.8503, -21.35) -> (352.8503, -21.35)
  line L829 (352.8503, -21.35) -> (352.8503, -24.35)
  line L830 (352.8503, -24.35) -> (349.8503, -24.35)
  line L831 (349.8503, -24.35) -> (349.8503, -21.35)
  line L832 (349.8503, -21.35) -> (346.8503, -21.35)
  line L833 (346.8503, -21.35) -> (346.8503, -24.35)
  line L834 (346.8503, -24.35) -> (343.8503, -24.35)
  line L835 (343.8503, -24.35) -> (343.8503, -21.35)
  line L836 (343.8503, -21.35) -> (340.8503, -21.35)
  line L837 (340.8503, -21.35) -> (340.8503, -24.35)
  line L838 (340.8503, -24.35) -> (337.8503, -24.35)
  line L839 (337.8503, -24.35) -> (337.8503, -21.35)
  line L840 (337.8503, -21.35) -> (334.8503, -21.35)
  line L841 (334.8503, -21.35) -> (334.8503, -24.35)
  line L842 (334.8503, -24.35) -> (331.8503, -24.35)
  line L843 (331.8503, -24.35) -> (331.8503, -21.35)
  line L844 (331.8503, -21.35) -> (327.1003, -21.35)
  line L845 (327.1003, -21.35) -> (327.1003, -24.35)
  line L846 (327.1003, -24.35) -> (322.3503, -24.35)
  line L847 (322.3503, -24.35) -> (322.3503, -20.6)
  line L848 (322.3503, -20.6) -> (325.3503, -20.6)
  line L849 (325.3503, -20.6) -> (325.3503, -16.85)
  line L850 (325.3503, -16.85) -> (322.3503, -16.85)
  line L851 (322.3503, -16.85) -> (322.3503, -13.85)
  line L852 (322.3503, -13.85) -> (325.3503, -13.85)
  line L853 (325.3503, -13.85) -> (325.3503, -10.1)
  line L854 (325.3503, -10.1) -> (322.3503, -10.1)
  line L855 (322.3503, -10.1) -> (322.3503, -6.35)
  line L856 (641.3505, -6.35) -> (642.1005, -6.35)
  line L857 (642.1005, -6.35) -> (642.1005, -9.35)
  line L858 (642.1005, -9.35) -> (645.8505, -9.35)
  line L859 (645.8505, -9.35) -> (645.8505, -6.35)
  line L860 (645.8505, -6.35) -> (648.8505, -6.35)
  line L861 (648.8505, -6.35) -> (648.8505, -9.35)
  line L862 (648.8505, -9.35) -> (651.8505, -9.35)
  line L863 (651.8505, -9.35) -> (651.8505, -6.35)
  line L864 (651.8505, -6.35) -> (654.8505, -6.35)
  line L865 (654.8505, -6.35) -> (654.8505, -9.35)
  line L866 (654.8505, -9.35) -> (657.8505, -9.35)
  line L867 (657.8505, -9.35) -> (657.8505, -6.35)
  line L868 (657.8505, -6.35) -> (660.8505, -6.35)
  line L869 (660.8505, -6.35) -> (660.8505, -9.35)
  line L870 (660.8505, -9.35) -> (663.8505, -9.35)
  line L871 (663.8505, -9.35) -> (663.8505, -6.35)
  line L872 (663.8505, -6.35) -> (666.8505, -6.35)
  line L873 (666.8505, -6.35) -> (666.8505, -9.35)
  line L874 (666.8505, -9.35) -> (669.8506, -9.35)
  line L875 (669.8506, -9.35) -> (669.8506, -6.35)
  line L876 (669.8506, -6.35) -> (672.8506, -6.35)
  line L877 (672.8506, -6.35) -> (672.8506, -9.35)
  line L878 (672.8506, -9.35) -> (675.8506, -9.35)
  line L879 (675.8506, -9.35) -> (675.8506, -6.35)
  line L880 (675.8506, -6.35) -> (678.8506, -6.35)
  line L881 (678.8506, -6.35) -> (678.8506, -9.35)
  line L882 (678.8506, -9.35) -> (681.8506, -9.35)
  line L883 (681.8506, -9.35) -> (681.8506, -6.35)
  line L884 (681.8506, -6.35) -> (684.8506, -6.35)
  line L885 (684.8506, -6.35) -> (684.8506, -9.35)
  line L886 (684.8506, -9.35) -> (687.8506, -9.35)
  line L887 (687.8506, -9.35) -> (687.8506, -6.35)
  line L888 (687.8506, -6.35) -> (690.8506, -6.35)
  line L889 (690.8506, -6.35) -> (690.8506, -9.35)
  line L890 (690.8506, -9.35) -> (693.8506, -9.35)
  line L891 (693.8506, -9.35) -> (693.8506, -6.35)
  line L892 (693.8506, -6.35) -> (696.8506, -6.35)
  line L893 (696.8506, -6.35) -> (696.8506, -9.35)
  line L894 (696.8506, -9.35) -> (699.8506, -9.35)
  line L895 (699.8506, -9.35) -> (699.8506, -6.35)
  line L896 (699.8506, -6.35) -> (702.8506, -6.35)
  line L897 (702.8506, -6.35) -> (702.8506, -9.35)
  line L898 (702.8506, -9.35) -> (705.8506, -9.35)
  line L899 (705.8506, -9.35) -> (705.8506, -6.35)
  line L900 (705.8506, -6.35) -> (708.8506, -6.35)
  line L901 (708.8506, -6.35) -> (708.8506, -9.35)
  line L902 (708.8506, -9.35) -> (711.8506, -9.35)
  line L903 (711.8506, -9.35) -> (711.8506, -6.35)
  line L904 (711.8506, -6.35) -> (714.8506, -6.35)
  line L905 (714.8506, -6.35) -> (714.8506, -9.35)
  line L906 (714.8506, -9.35) -> (717.8506, -9.35)
  line L907 (717.8506, -9.35) -> (717.8506, -6.35)
  line L908 (717.8506, -6.35) -> (720.8506, -6.35)
  line L909 (720.8506, -6.35) -> (720.8506, -9.35)
  line L910 (720.8506, -9.35) -> (723.8506, -9.35)
  line L911 (723.8506, -9.35) -> (723.8506, -6.35)
  line L912 (723.8506, -6.35) -> (726.8506, -6.35)
  line L913 (726.8506, -6.35) -> (726.8506, -9.35)
  line L914 (726.8506, -9.35) -> (729.8506, -9.35)
  line L915 (729.8506, -9.35) -> (729.8506, -6.35)
  line L916 (729.8506, -6.35) -> (732.8506, -6.35)
  line L917 (732.8506, -6.35) -> (732.8506, -9.35)
  line L918 (732.8506, -9.35) -> (735.8506, -9.35)
  line L919 (735.8506, -9.35) -> (735.8506, -6.35)
  line L920 (735.8506, -6.35) -> (738.8506, -6.35)
  line L921 (738.8506, -6.35) -> (738.8506, -9.35)
  line L922 (738.8506, -9.35) -> (741.8506, -9.35)
  line L923 (741.8506, -9.35) -> (741.8506, -6.35)
  line L924 (741.8506, -6.35) -> (744.8506, -6.35)
  line L925 (744.8506, -6.35) -> (744.8506, -9.35)
  line L926 (744.8506, -9.35) -> (747.8506, -9.35)
  line L927 (747.8506, -9.35) -> (747.8506, -6.35)
  line L928 (747.8506, -6.35) -> (750.8506, -6.35)
  line L929 (750.8506, -6.35) -> (750.8506, -9.35)
  line L930 (750.8506, -9.35) -> (753.8506, -9.35)
  line L931 (753.8506, -9.35) -> (753.8506, -6.35)
  line L932 (753.8506, -6.35) -> (756.8506, -6.35)
  line L933 (756.8506, -6.35) -> (756.8506, -9.35)
  line L934 (756.8506, -9.35) -> (759.8506, -9.35)
  line L935 (759.8506, -9.35) -> (759.8506, -6.35)
  line L936 (759.8506, -6.35) -> (762.8506, -6.35)
  line L937 (762.8506, -6.35) -> (762.8506, -9.35)
  line L938 (762.8506, -9.35) -> (765.8506, -9.35)
  line L939 (765.8506, -9.35) -> (765.8506, -6.35)
  line L940 (765.8506, -6.35) -> (768.8506, -6.35)
  line L941 (768.8506, -6.35) -> (768.8506, -9.35)
  line L942 (768.8506, -9.35) -> (771.8506, -9.35)
  line L943 (771.8506, -9.35) -> (771.8506, -6.35)
  line L944 (771.8506, -6.35) -> (774.8506, -6.35)
  line L945 (774.8506, -6.35) -> (774.8506, -9.35)
  line L946 (774.8506, -9.35) -> (777.8506, -9.35)
  line L947 (777.8506, -9.35) -> (777.8506, -6.35)
  line L948 (777.8506, -6.35) -> (780.8506, -6.35)
  line L949 (780.8506, -6.35) -> (780.8506, -9.35)
  line L950 (780.8506, -9.35) -> (783.8506, -9.35)
  line L951 (783.8506, -9.35) -> (783.8506, -6.35)
  line L952 (783.8506, -6.35) -> (786.8506, -6.35)
  line L953 (786.8506, -6.35) -> (786.8506, -9.35)
  line L954 (786.8506, -9.35) -> (790.6007, -9.35)
  line L955 (790.6007, -9.35) -> (790.6007, -6.35)
  line L956 (790.6007, -6.35) -> (791.3507, -6.35)
  line L957 (791.3507, -6.35) -> (791.3507, -10.1)
  line L958 (791.3507, -10.1) -> (794.3507, -10.1)
  line L959 (794.3507, -10.1) -> (794.3507, -13.85)
  line L960 (794.3507, -13.85) -> (791.3507, -13.85)
  line L961 (791.3507, -13.85) -> (791.3507, -16.85)
  line L962 (791.3507, -16.85) -> (794.3507, -16.85)
  line L963 (794.3507, -16.85) -> (794.3507, -20.6)
  line L964 (794.3507, -20.6) -> (791.3507, -20.6)
  line L965 (791.3507, -20.6) -> (791.3507, -24.35)
  line L966 (791.3507, -24.35) -> (790.6007, -24.35)
  line L967 (790.6007, -24.35) -> (790.6007, -21.35)
  line L968 (790.6007, -21.35) -> (786.8506, -21.35)
  line L969 (786.8506, -21.35) -> (786.8506, -24.35)
  line L970 (786.8506, -24.35) -> (783.8506, -24.35)